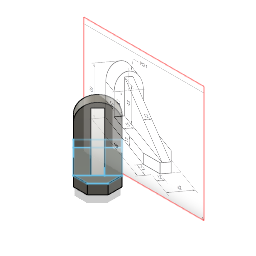
A1 (Autodesk Fusion 360 design; units mm, degrees)
Autodesk Fusion 360 part; units mm, degrees
sketch "Sketch1" plane through (0, 0, 0) normal (0, 1, 0) x (1, 0, 0)
  line L0 (-51.0653, -15.1777) -> (-12.8816, -53.3615)
  line L1 (-12.8816, -53.3615) -> (4.089, -53.3615)
  line L2 (4.089, -53.3615) -> (16.8169, -40.6336)
  line L3 (16.8169, -40.6336) -> (16.8169, -23.663)
  line L4 (16.8169, -23.663) -> (-21.3669, 14.5207)
  line L5 (-21.3669, 14.5207) -> (-51.0653, -15.1777)
  line L6 (-12.8816, -53.3615) -> (16.8169, -23.663)
  line L7 (-40.4587, -4.5711) -> (-2.275, -42.7549)
  line L8 (-31.9735, 3.9141) -> (6.2103, -34.2696)
  line L9 (-42.5801, -23.663) -> (-12.8816, 6.0355)
  dimension "d2" = 66
  dimension "d3" = 12
  dimension "d4" = 18
  dimension "d5" = 42
  dimension "d6" = 15
  dimension "d7" = 15
  dimension "d10" = 12
  dimension "d11" = 12
  constraint horizontal L1
  constraint perpendicular L1 L3
  constraint parallel L0 L4
  constraint equal L0 L4
  constraint parallel L2 L5
  constraint equal L1 L3
  constraint coincident L5 L7.start
  constraint coincident L6 L7.end
  constraint perpendicular L6 L7
  constraint coincident L5 L8.start
  constraint coincident L6 L8.end
  constraint parallel L0 L7
  constraint parallel L7 L8
  constraint coincident L0 L9.start
  constraint coincident L4 L9.end
  constraint parallel L5 L9
  measures "d2" distance of L2 L5
  measures "d3" distance of L2 L6
  measures "d4" distance of L1.end L2.end
  measures "d5" distance of L0.start L4.end
  measures "d6" distance of L0 L7
  measures "d7" distance of L4 L8
  measures "d10" distance of L7 L8
  measures "d11" distance of L0.start L9.start
extrude "Extrude1" add sketch "Sketch1" against normal blind 12 makes body 1
extrude "Extrude2" add sketch "Sketch1" along normal blind 27 separate body contours L0 L5 L7 L9 | L5 L7 L8 L9 | L4 L5 L8 L9 makes body 2
extrude "Extrude3" add sketch "Sketch1" along normal blind 42 contours L6 L7 L8 L9 bodies 2
draft "Draft1" angle -45 neutral plane through (-31.9735, 0, 13.0564) pull (-0.707107, 0, -0.707107) 1 faces at (-6.5176, 42, 27.1986) on bodies 2
extrude "Extrude4" add 1 faces at (-34.8019, 27, 4.5711) along direction (0, 1, 0) blind 21 separate body on bodies 2 makes body 3
fillet "Fillet1" radius 21 1 edges at (-46.8227, 48, 19.4204) on bodies 3
fillet "Fillet2" radius 21 1 edges at (-17.1242, 48, -10.2781) on bodies 3
combine "Combine1" operation add target body 1 tool bodies 2 3
equation "d4 = 42 mm - 24 mm"
equation "d20 = 60 mm - 12 mm - 27 mm"
named bodies: "A1"
